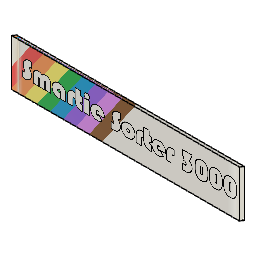
name_sign (Autodesk Fusion 360 design; units mm, degrees)
Autodesk Fusion 360 part; units mm, degrees
sketch "Name Sign" plane through (0, 0, 0) normal (1, 0, 0) x (0, 1, 0) in component "Name Sign"
  line L0 (-0.0158, 97.2466) -> (5.9842, 94.7858)
  line L1 (5.9842, 150.2078) -> (-0.0158, 152.6686)
  line L2 (-0.0158, 152.6686) -> (-0.0158, 97.2466)
  line L3 (5.9842, 150.2078) -> (5.9842, 94.7858)
  dimension "d18" = 67.7
  dimension "d8" = 6
  dimension "d9" = 55.422
  constraint vertical L2
  constraint parallel L2 L3
  measures "d18" angle of L0 L3
  measures "d8" distance of L2 L3
  measures "d9" distance of L1.end L0.start
extrude "Extrude2" add sketch "Name Sign" along normal blind 270 in component "Name Sign"
component "Name Sign" placed x (1, 0, 0) y (0, 1, 0) z (0, 0, 1) at (0, 0, 0)
equation "polycarbonateThickness = 6 mm" comment "Thickness of the polycarbonate panels"
named bodies: "Name Sign"
